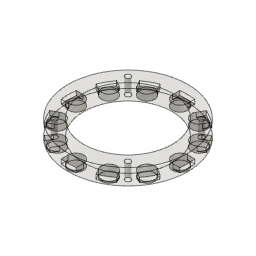
machining-setup v2_machining-setup 3DP v4 (Autodesk Fusion 360 design; units mm, degrees)
Autodesk Fusion 360 part; units mm, degrees
sketch "Sketch1" plane through (0, 0, 9.525) normal (0, 0, 1) x (-1, 0, 0) in component "magnet holder"
  arc A0 (0, -47.625) -> (-95.25, -47.625) centre (-47.625, -47.625) ccw
  line L0 (-95.25, -47.625) -> (-95.25, -130.175)
  arc A1 (-95.25, -130.175) -> (0, -130.175) centre (-47.625, -130.175) ccw
  line L1 (0, -130.175) -> (0, -47.625)
  circle A2 centre (-47.625, -130.175) radius 35.306
  circle A3 centre (-47.625, -130.175) radius 47.625
  circle A4 centre (-47.625, -130.175) radius 35.306
  circle A5 centre (-47.625, -41.275) radius 39.37
  circle A6 centre (-18.3045, -159.4955) radius 2.159
  circle A7 centre (-76.9455, -159.4955) radius 2.159
  circle A8 centre (-18.3045, -100.8545) radius 2.159
  circle A9 centre (-76.9455, -100.8545) radius 2.159
  dimension "d96_1" = 4.318
  dimension "d97_1" = 4.318
  dimension "d98_1" = 4.318
  dimension "d99_1" = 4.318
  constraint concentric A1 A3
  constraint concentric A3 A4
  measures "d96_1" diameter of A6
  measures "d97_1" diameter of A7
  measures "d98_1" diameter of A8
  measures "d99_1" diameter of A9
extrude "Extrude1" add sketch "Sketch1" along normal blind 5.588 contours A1 A3 in component "magnet holder"
sketch "Sketch2" plane through (0, 0, 9.525) normal (0, 0, -1) x (1, 0, 0) in component "magnet holder"
  circle A0 centre (47.625, -130.175) radius 35.306
  circle A1 centre (47.625, -130.175) radius 47.625
  circle A2 centre (47.625, -130.175) radius 41.4655 construction
  circle A3 centre (47.625, -88.7095) radius 6
  circle A4 centre (26.8922, -94.2648) radius 6
  circle A5 centre (11.7148, -109.4422) radius 6
  circle A6 centre (6.1595, -130.175) radius 6
  circle A7 centre (11.7148, -150.9077) radius 6
  circle A8 centre (26.8922, -166.0852) radius 6
  circle A9 centre (47.625, -171.6405) radius 6
  circle A10 centre (68.3577, -166.0852) radius 6
  circle A11 centre (83.5352, -150.9078) radius 6
  circle A12 centre (89.0905, -130.175) radius 6
  circle A13 centre (83.5352, -109.4423) radius 6
  circle A14 centre (68.3578, -94.2648) radius 6
  circle A15 centre (76.9455, -100.8545) radius 2.159
  circle A16 centre (18.3045, -100.8545) radius 2.159
  circle A17 centre (18.3045, -159.4955) radius 2.159
  circle A18 centre (76.9455, -159.4955) radius 2.159
  dimension "d91_1" = 12
  dimension "d93_1" = 360
  constraint concentric A0 A2
  constraint coincident A2 A3.centre
  measures "d91_1" diameter of A3
extrude "Extrude2" cut sketch "Sketch2" against normal blind 4.0005 contours A3 | A4 | A5 | A6 | A7 | A8 | A9 | A10 | A11 | A12 | A13 | A14 in component "magnet holder"
sketch "Sketch1 (2)" plane through (0, 0, 15.875) normal (0, 0, 1) x (-1, 0, 0) in component "magnet spacer"
  circle A0 centre (-76.9455, -100.8545) radius 1.651
  circle A1 centre (-18.3045, -100.8545) radius 1.651
  circle A2 centre (-18.3045, -159.4955) radius 1.651
  circle A3 centre (-76.9455, -159.4955) radius 1.651
  circle A4 centre (-47.625, -130.175) radius 35.306
  circle A5 centre (-47.625, -130.175) radius 47.625
  circle A6 centre (-47.625, -130.175) radius 47.625
  circle A7 centre (-18.3045, -159.4955) radius 1.651
  circle A8 centre (-76.9455, -159.4955) radius 1.651
  circle A9 centre (-76.9455, -100.8545) radius 1.651
  circle A10 centre (-18.3045, -100.8545) radius 1.651
  constraint concentric A4 A6
  constraint concentric A2 A7
  constraint concentric A3 A8
  constraint concentric A0 A9
  constraint concentric A1 A10
sketch "Sketch1 (3)" plane through (0, 0, 16.6622) normal (0, 0, 1) x (-1, 0, 0)
  circle A0 centre (-11.7148, -109.4423) radius 6
  circle A1 centre (-83.5352, -150.9077) radius 6
  circle A2 centre (-11.7148, -150.9078) radius 6
  circle A3 centre (-6.1595, -130.175) radius 6
  circle A4 centre (-89.0905, -130.175) radius 6
  circle A5 centre (-26.8922, -94.2648) radius 6
  circle A6 centre (-68.3577, -94.2648) radius 6
  circle A7 centre (-68.3577, -166.0852) radius 6
  circle A8 centre (-26.8922, -166.0852) radius 6
  circle A9 centre (-47.625, -171.6405) radius 6
  circle A10 centre (-83.5352, -109.4422) radius 6
  circle A11 centre (-47.625, -88.7095) radius 6
  circle A12 centre (-76.9455, -159.4955) radius 2.159
  circle A13 centre (-47.625, -130.175) radius 35.306
  circle A14 centre (-76.9455, -100.8545) radius 2.159
  circle A15 centre (-18.3045, -159.4955) radius 2.159
  circle A16 centre (-18.3045, -100.8545) radius 2.159
  circle A17 centre (-47.625, -130.175) radius 47.625
  line L0 (-53.625, -88.7095) -> (-53.625, -82.8628)
  line L1 (-41.6392, -89.1226) -> (-41.6392, -82.7277)
  line L2 (-73.5539, -97.2648) -> (-76.4772, -92.2015)
  line L3 (-62.9674, -91.6297) -> (-66.1648, -86.0915)
  line L4 (-86.5352, -114.6384) -> (-91.5985, -111.7151)
  line L5 (-80.1845, -104.465) -> (-85.7227, -101.2675)
  line L6 (-89.0905, -136.175) -> (-94.9372, -136.175)
  line L7 (-88.6774, -124.1892) -> (-95.0723, -124.1892)
  line L8 (-80.5352, -156.1039) -> (-85.5985, -159.0272)
  line L9 (-86.1703, -145.5174) -> (-91.7085, -148.7148)
  line L10 (-63.1616, -169.0852) -> (-66.0849, -174.1485)
  line L11 (-73.335, -162.7345) -> (-76.5325, -168.2727)
  line L12 (-41.625, -171.6405) -> (-41.625, -177.4872)
  line L13 (-53.6108, -171.2274) -> (-53.6108, -177.6223)
  line L14 (-21.6961, -163.0852) -> (-18.7728, -168.1485)
  line L15 (-32.2826, -168.7203) -> (-29.0852, -174.2585)
  line L16 (-8.7148, -145.7116) -> (-3.6515, -148.6349)
  line L17 (-15.0655, -155.885) -> (-9.5273, -159.0825)
  line L18 (-6.1595, -124.175) -> (-0.3128, -124.175)
  line L19 (-6.5726, -136.1608) -> (-0.1777, -136.1608)
  line L20 (-14.7148, -104.2461) -> (-9.6515, -101.3228)
  line L21 (-9.0797, -114.8326) -> (-3.5415, -111.6352)
  line L22 (-32.0884, -91.2648) -> (-29.1651, -86.2015)
  line L23 (-21.915, -97.6155) -> (-18.7175, -92.0773)
  point P0 (-53.625, -88.7095)
  dimension "d2" = 360
  constraint coincident P0 L0.start
  constraint vertical L0
  constraint coincident A11 L1.start
  constraint vertical L1
extrude "Extrude3" cut sketch "Sketch1 (3)" against normal blind 3.5 contours A0 A17 L20 L21 | A5 A17 L22 L23 | A3 A17 L18 L19 | A11 A17 L0 L1 | A2 A17 L16 L17 | A6 A17 L2 L3 | A8 A17 L14 L15 | A10 A17 L4 L5 | A9 A17 L12 L13 | A4 A17 L6 L7 | A7 A17 L10 L11 | A1 A17 L8 L9 sketch seen with x (-1, 0, 0) y (0, 1, 0) z (0, 0, -1) at (95.25, 0, 26.1872) in component "magnet holder"
sketch "Sketch2 (2)" plane through (0, 0, 16.6622) normal (0, 0, 1) x (-1, 0, 0)
  line L0 (-80.5352, -156.1039) -> (-85.5408, -158.9939)
  arc A0 (-85.5408, -158.9939) -> (-76.4325, -168.0995) centre (-47.625, -130.175) ccw
  line L1 (-76.4325, -168.0995) -> (-73.7481, -163.4501)
  arc A1 (-63.1616, -169.0852) -> (-73.7481, -163.4501) centre (-68.3577, -166.0852) ccw
  line L2 (-63.1616, -169.0852) -> (-66.0516, -174.0908)
  arc A2 (-66.0516, -174.0908) -> (-53.6108, -177.4223) centre (-47.625, -130.175) ccw
  line L3 (-53.6108, -177.4223) -> (-53.6108, -172.0536)
  arc A3 (-41.625, -171.6405) -> (-53.6108, -172.0536) centre (-47.625, -171.6405) ccw
  line L4 (-41.625, -171.6405) -> (-41.625, -177.4205)
  arc A4 (-41.625, -177.4205) -> (-29.1852, -174.0853) centre (-47.625, -130.175) ccw
  line L5 (-29.1852, -174.0853) -> (-31.8695, -169.4358)
  arc A5 (-21.6961, -163.0852) -> (-31.8695, -169.4358) centre (-26.8922, -166.0852) ccw
  line L6 (-21.6961, -163.0852) -> (-18.8061, -168.0908)
  arc A6 (-18.8061, -168.0908) -> (-9.7005, -158.9825) centre (-47.625, -130.175) ccw
  line L7 (-9.7005, -158.9825) -> (-14.3499, -156.2981)
  arc A7 (-8.7148, -145.7116) -> (-14.3499, -156.2981) centre (-11.7148, -150.9078) ccw
  line L8 (-8.7148, -145.7116) -> (-3.7092, -148.6016)
  arc A8 (-3.7092, -148.6016) -> (-0.3777, -136.1608) centre (-47.625, -130.175) ccw
  line L9 (-0.3777, -136.1608) -> (-5.7464, -136.1608)
  arc A9 (-6.1595, -124.175) -> (-5.7464, -136.1608) centre (-6.1595, -130.175) ccw
  line L10 (-6.1595, -124.175) -> (-0.3795, -124.175)
  arc A10 (-0.3795, -124.175) -> (-3.7147, -111.7352) centre (-47.625, -130.175) ccw
  line L11 (-3.7147, -111.7352) -> (-8.3642, -114.4195)
  arc A11 (-14.7148, -104.2461) -> (-8.3642, -114.4195) centre (-11.7148, -109.4423) ccw
  line L12 (-14.7148, -104.2461) -> (-9.7092, -101.3561)
  arc A12 (-9.7092, -101.3561) -> (-18.8175, -92.2505) centre (-47.625, -130.175) ccw
  line L13 (-18.8175, -92.2505) -> (-21.5019, -96.8999)
  arc A13 (-32.0884, -91.2648) -> (-21.5019, -96.8999) centre (-26.8922, -94.2648) ccw
  line L14 (-32.0884, -91.2648) -> (-29.1984, -86.2592)
  arc A14 (-29.1984, -86.2592) -> (-41.6392, -82.9277) centre (-47.625, -130.175) ccw
  line L15 (-41.6392, -82.9277) -> (-41.6392, -88.2964)
  arc A15 (-53.625, -88.7095) -> (-41.6392, -88.2964) centre (-47.625, -88.7095) ccw
  line L16 (-53.625, -88.7095) -> (-53.625, -82.9295)
  arc A16 (-53.625, -82.9295) -> (-66.0648, -86.2647) centre (-47.625, -130.175) ccw
  line L17 (-66.0648, -86.2647) -> (-63.3805, -90.9142)
  arc A17 (-73.5539, -97.2648) -> (-63.3805, -90.9142) centre (-68.3577, -94.2648) ccw
  line L18 (-73.5539, -97.2648) -> (-76.4439, -92.2592)
  arc A18 (-76.4439, -92.2592) -> (-85.5495, -101.3675) centre (-47.625, -130.175) ccw
  line L19 (-85.5495, -101.3675) -> (-80.9001, -104.0519)
  arc A19 (-86.5352, -114.6384) -> (-80.9001, -104.0519) centre (-83.5352, -109.4422) ccw
  line L20 (-86.5352, -114.6384) -> (-91.5408, -111.7484)
  arc A20 (-91.5408, -111.7484) -> (-94.8723, -124.1892) centre (-47.625, -130.175) ccw
  line L21 (-94.8723, -124.1892) -> (-89.5036, -124.1892)
  arc A21 (-89.0905, -136.175) -> (-89.5036, -124.1892) centre (-89.0905, -130.175) ccw
  line L22 (-89.0905, -136.175) -> (-94.8705, -136.175)
  arc A22 (-94.8705, -136.175) -> (-91.5353, -148.6148) centre (-47.625, -130.175) ccw
  line L23 (-91.5353, -148.6148) -> (-86.8858, -145.9305)
  arc A23 (-80.5352, -156.1039) -> (-86.8858, -145.9305) centre (-83.5352, -150.9077) ccw
  circle A24 centre (-76.9455, -159.4955) radius 2.159
  circle A25 centre (-47.625, -130.175) radius 35.306
  circle A26 centre (-76.9455, -100.8545) radius 2.159
  circle A27 centre (-18.3045, -159.4955) radius 2.159
  circle A28 centre (-18.3045, -100.8545) radius 2.159
  circle A29 centre (-47.625, -130.175) radius 47.625
  circle A30 centre (-47.625, -130.175) radius 35.306
  constraint concentric A0 A29
  constraint concentric A29 A30
extrude "Extrude4" add sketch "Sketch2 (2)" along normal blind 7.112 sketch seen with x (-1, 0, 0) y (0, 1, 0) z (0, 0, -1) at (95.25, 0, 26.1872) in component "magnet holder"
extrude "Extrude5" cut 12 faces at (67.6271, 167.9469, 13.5255) (80.8432, 151.7755, 13.5255) (89.6447, 133.5821, 13.5255) (81.9802, 105.2788, 13.5255) (67.3578, 90.2795, 13.5255) (49.4935, 89.8687, 13.5255) (28.8699, 95.1458, 13.5255) (10.1395, 112.2599, 13.5255) (6.6045, 131.9486, 13.5255) (10.9841, 149.046, 13.5255) (26.1616, 167.9469, 13.5255) (50.8883, 170.7727, 13.5255) along direction (0, 0, 1) blind 0.8382 in component "magnet holder"
component "magnet holder" placed x (-1, 0, 0) y (0, 1, 0) z (0, 0, -1) at (95.25, 0, 26.1872)
component "magnet spacer" placed x (1, 0, 0) y (0, 1, 0) z (0, 0, 1) at (0, 104.14, -5.5626)
equation "d91_1 = ( 12 / 25.4 ) * 1 in"
equation "d94_1 = ( -3 / 16 ) * 1 in + 0.03 in"
equation "d101_1 = 0.0 deg"
equation "d3 = ( -3.5 / 25.4 ) * 1 in"
equation "d5 = 0.5 in - 0.22 in"
